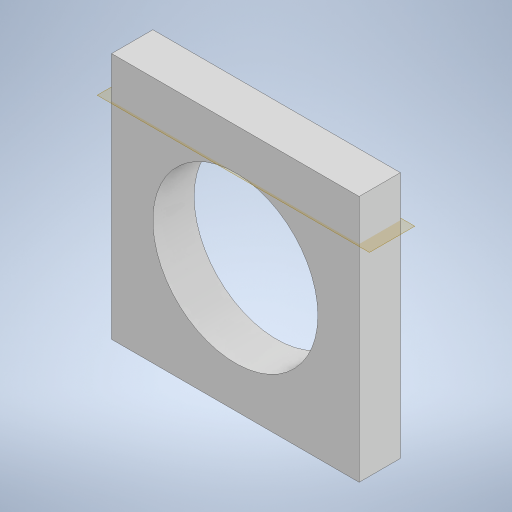
# Autodesk Inventor part: AGUJERO
Saved by Autodesk Inventor 2023.2 (Build 272271030, 271C)
## iProperties
Created: 2023-10-02
Part Number: AGUJERO
Material: Generic
Document SubType Name: Modeling
Designer: Cris Pat
Density: 1 g/cm^3
Appearance: Default
Author: Cris Pat
Autodesk Inventor part; units mm, degrees
ref_plane "YZ Plane" through (0, 0, 0) normal (1, 0, 0) x (0, 1, 0)
ref_plane "XY Plane" through (0, 0, 0) normal (0, 0, 1) x (1, 0, 0)
sketch "Sketch1" plane through (0, 0, 0) normal (0, 0, 1) x (1, 0, 0)
  line L0 (-150, -150) -> (150, -150)
  line L1 (150, -150) -> (150, 150)
  line L2 (150, 150) -> (-150, 150)
  line L3 (-150, 150) -> (-150, -150)
  line L4 (-150, -150) -> (150, 150) construction
  line L5 (150, -150) -> (-150, 150) construction
  point P0 (0, 0)
  dimension "d0" = 300
  dimension "d1" = 300
  constraints: 12 end point, 2 midpoint, 2 parallel, 1 horizontal, 1 perpendicular
  measures "d0" distance of L2.end L1.end
  measures "d1" distance of L1.end L0.end
extrude "Extrusion1" add sketch "Sketch1" along normal blind 50
sketch "Sketch2" plane through (0, 0, 50) normal (0, 0, 1) x (1, 0, 0)
  circle A0 centre (0, 0) radius 100.0115
  dimension "D_agujero" = 200
  constraints: 1 centre point, 1 coincident
extrude "Extrusion2" cut sketch "Sketch2" against normal through all
ref_plane "Work Plane1" through (0, 100.0115, 50) normal (0, 1, 0) x (-1, 0, 0)
equation "\"d0\" = 1.5 * tamanio_basico"
equation "\"d1\" = 1.5 * tamanio_basico"
equation "\"espesor\" = 0.25 * tamanio_basico"
equation "\"D_agujero\" = tamanio_basico"
equation "\"tamanio_basico\" = 200"
body "Solid1"
